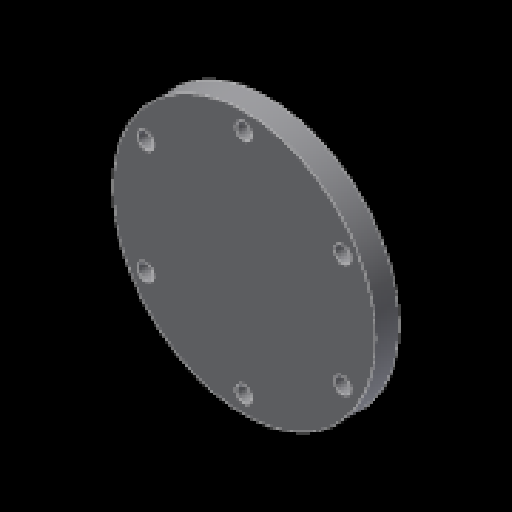
# Autodesk Inventor part: LegEncoderHub
Saved by Autodesk Inventor 2025.2 (Build 292293000, 293)
## iProperties
Created: 2025-10-14
Part Number: LegEncoderHub
Material: Generic
Document SubType Name: Sheet Metal
Designer: valer
Density: 1 g/cm^3
Appearance: Default
Sheet Metal Rule: Default
Author: valer
Autodesk Inventor part; units mm, degrees
ref_plane "YZ Plane" through (0, 0, 0) normal (1, 0, 0) x (0, 1, 0)
ref_plane "XZ Plane" through (0, 0, 0) normal (0, 1, 0) x (-1, 0, 0)
ref_plane "XY Plane" through (0, 0, 0) normal (0, 0, 1) x (1, 0, 0)
sketch "Base" plane through (0, 0, 0) normal (0, 0, 1) x (1, 0, 0)
  circle A0 centre (14.2875, 0) radius 14.2875 construction
  circle A1 centre (34.9097, 11.9062) radius 1.9939 construction
  circle A2 centre (34.9097, -11.9063) radius 1.9939 construction
  circle A3 centre (14.2875, -23.8125) radius 1.9939 construction
  circle A4 centre (-6.3347, -11.9062) radius 1.9939 construction
  circle A5 centre (-6.3347, 11.9063) radius 1.9939 construction
  circle A6 centre (14.2875, 23.8125) radius 1.9939 construction
  circle A7 centre (14.2875, 0) radius 27.5127
  arc A8 (34.1709, -15.825) -> (37.934, -9.307) centre (34.9097, -11.9063) ccw construction
  circle A9 centre (-6.3347, 11.9063) radius 1.7272
  circle A10 centre (14.2875, 23.8125) radius 1.7272
  circle A11 centre (34.9097, 11.9062) radius 1.7272
  circle A12 centre (34.9097, -11.9063) radius 1.7272
  circle A13 centre (14.2875, -23.8125) radius 1.7272
  circle A14 centre (-6.3347, -11.9062) radius 1.7272
  point P0 (0, 0)
  dimension "d3" = 55.0254
  dimension "d10" = 3.4544
  constraints: 7 centre point, 7 coincident, 5 equal radius, 1 horizontal alignment
  measures "d3" diameter of A7
  measures "d10" diameter of A9
extrude "BaseFeature" add sketch "Base" along normal blind 5
sketch "WheelMagnetAlignmentFlangeMountHoles" plane through (14.2875, 0, 0) normal (0, 0, -1) x (-1, 0, 0)
  circle A0 centre (4.5, 4.5) radius 1.225 projected
  circle A1 centre (4.5, -4.5) radius 1.225 projected
  circle A2 centre (-4.5, -4.5) radius 1.225 projected
  circle A3 centre (-4.5, 4.5) radius 1.225 projected
  point P0 (14.2875, 0)
extrude "Cut1" cut sketch "WheelMagnetAlignmentFlangeMountHoles" against normal blind 3.048
equation "\"d45\" = Thickness"
equation "\"BendRadius\" = Thickness"
equation "\"BendReliefWidth\" = Thickness"
equation "\"BendReliefDepth\" = 0.5 * Thickness"
equation "\"CornerReliefSize\" = 4 * Thickness"
equation "\"MinimumRemnant\" = 2 * Thickness"
equation "\"TransitionRadius\" = BendRadius"
equation "\"JacobiRadiusSize\" = BendRadius"
equation "\"GapSize\" = Thickness"
equation "\"d44\" = Thickness"
equation "\"Thickness\" = 3.048"
body "Solid1"
